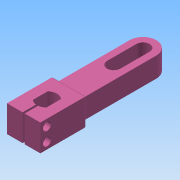
# Autodesk Inventor part: 刀轴拨叉
Saved by Autodesk Inventor 2015 (Build 190159000, 159)
## iProperties
Created: 2017-05-26
Part Number: 刀轴拨叉
Material: 常规
Document SubType Name: Modeling
Designer: Administrator
Density: 1 g/cm^3
Appearance: 粉红色
Author: Administrator
Autodesk Inventor part; units mm, degrees
ref_plane "YZ Plane" through (0, 0, 0) normal (1, 0, 0) x (0, 1, 0)
ref_plane "XZ Plane" through (0, 0, 0) normal (0, 1, 0) x (-1, 0, 0)
ref_plane "XY Plane" through (0, 0, 0) normal (0, 0, 1) x (1, 0, 0)
sketch "草图1" plane through (0, 0, 0) normal (0, 0, 1) x (1, 0, 0)
  line L0 (-12.5, 17.5) -> (12.5, 17.5)
  line L1 (12.5, 17.5) -> (12.5, -17.5)
  line L2 (12.5, -17.5) -> (-12.5, -17.5)
  line L3 (-12.5, -17.5) -> (-12.5, 17.5)
  line L4 (0, 0) -> (12.5, 0)
  line L5 (0, 0) -> (0, 17.5)
  circle A0 centre (0, 0) radius 7.5
  line L6 (10, 17.5) -> (-10, 17.5)
  line L7 (-10, 17.5) -> (-10, 82)
  line L8 (-10, 82) -> (10, 82)
  line L9 (10, 82) -> (10, 17.5)
  point P0 (0, 82)
  dimension "d0" = 25
  dimension "d1" = 35
  dimension "d2" = 15
  dimension "d3" = 20
  dimension "d13" = 82
  constraints: 20 end point, 5 parallel, 3 horizontal, 3 midpoint, 2 perpendicular, 2 point on line, 1 centre point, 1 coincident
  measures "d0" distance of L1.end L2.end
  measures "d1" distance of L0.end L1.end
  measures "d2" diameter of A0
  measures "d3" distance of L7.end L8.end
  measures "d13" distance from line of L4.start L8
extrude "拉伸1" add sketch "草图1" along normal blind 20
sketch "草图2" plane through (0, 0, 20) normal (0, 0, 1) x (1, 0, 0)
  circle A0 centre (0, 0) radius 7.5
  line L0 (-12.5, -17.5) -> (12.5, -17.5) projected
  line L1 (-0.75, -7.4624) -> (0.75, -7.4624)
  line L2 (0.75, -7.4624) -> (0.75, -17.5)
  line L3 (0.75, -17.5) -> (-0.75, -17.5)
  line L4 (-0.75, -17.5) -> (-0.75, -7.4624)
  circle A1 centre (0, 72) radius 5
  circle A2 centre (0, 50) radius 5
  line L5 (10, 82) -> (-10, 82) projected
  line L6 (-5, 72) -> (-5, 50)
  line L7 (5, 72) -> (5, 50)
  line L8 (10, 17.5) -> (10, 82) projected
  dimension "d7" = 15
  dimension "d8" = 1.5
  dimension "d9" = 10
  dimension "d10" = 10
  dimension "d11" = 10
  dimension "d12" = 50
  dimension "d14" = 10
  constraints: 12 end point, 6 point on circle, 4 tangent, 3 centre point, 2 parallel, 1 coincident, 1 horizontal, 1 perpendicular, 1 point on line, 1 vertical
  measures "d7" diameter of A0
  measures "d8" distance between parallel lines of L2 L4
  measures "d9" diameter of A1
  measures "d10" diameter of A2
  measures "d11" distance from line of L5 A1.centre
  measures "d12" distance of point (0, 0) A2.centre
  measures "d14" distance from line of L8 A1.centre
extrude "拉伸2" cut sketch "草图2" against normal through all
sketch "草图3" plane through (10, 17.5, 0) normal (1, 0, 0) x (0, 0, -1)
  line L0 (0, 0) -> (-20, 0) projected
  line L1 (-20, 64.5) -> (-17.5, 64.5)
  line L2 (-17.5, 64.5) -> (-17.5, 0)
  line L3 (-17.5, 0) -> (-20, 0)
  line L4 (-20, 0) -> (-20, 64.5)
  line L5 (0, 64.5) -> (-2.5, 64.5)
  line L6 (-2.5, 64.5) -> (-2.5, 0)
  line L7 (-2.5, 0) -> (0, 0)
  line L8 (0, 0) -> (0, 64.5)
  point P0 (0, -17.5)
  dimension "d17" = 15
  dimension "d18" = 2.5
  constraints: 16 end point, 4 parallel, 2 horizontal, 2 perpendicular, 2 point on line
  measures "d17" distance between parallel lines of L6 L2
  measures "d18" distance between parallel lines of L4 L2
extrude "拉伸3" cut sketch "草图3" against normal through all
sketch "草图4" plane through (-12.5, -17.5, 0) normal (-1, 0, 0) x (0, 0, 1)
  circle A0 centre (5, 5) radius 1.5
  circle A1 centre (15, 5) radius 1.5
  line L0 (0, 0) -> (20, 0) projected
  line L1 (20, 35) -> (20, 0) projected
  line L2 (0, 35) -> (0, 0) projected
  point P0 (0, 17.5)
  dimension "d21" = 3
  dimension "d22" = 3
  dimension "d23" = 5
  dimension "d24" = 5
  dimension "d25" = 5
  dimension "d26" = 5
  constraints: 2 centre point
  measures "d21" diameter of A0
  measures "d22" diameter of A1
  measures "d23" distance from line of L0 A1.centre
  measures "d24" distance from line of L0 A0.centre
  measures "d25" distance from line of L1 A1.centre
  measures "d26" distance from line of L2 A0.centre
extrude "拉伸4" cut sketch "草图4" against normal through all
sketch "草图5" plane through (12.5, -17.5, 0) normal (1, 0, 0) x (0, 0, -1)
  circle A0 centre (-5, 5) radius 3
  circle A1 centre (-15, 5) radius 3
  circle A2 centre (-5, 5) radius 1.5 projected
  circle A3 centre (-15, 5) radius 1.5 projected
  point P0 (0, 17.5)
  dimension "d29" = 6
  dimension "d30" = 6
  constraints: 2 centre point, 2 concentric
  measures "d29" diameter of A0
  measures "d30" diameter of A1
extrude "拉伸5" cut sketch "草图5" against normal blind 4
thread "螺纹1" size "M3x0.5" class "6H" standard "ANSI Metric M Profile" full length
thread "螺纹2" size "M3x0.5" class "6H" standard "ANSI Metric M Profile" full length
sketch "草图6" plane through (0, 0, 0) normal (0, 0, -1) x (-1, 0, 0)
  line L0 (5, 5.5902) -> (5, -5.5902)
  line L1 (5, -5.5902) -> (-5, -5.5902)
  line L2 (-5, -5.5902) -> (-5, 5.5902)
  arc A0 (0.75, -7.4624) -> (-0.75, -7.4624) centre (0, 0) ccw projected
  arc A1 (-5, 5.5902) -> (-5, -5.5902) centre (0, 0) ccw
  arc A2 (5, -5.5902) -> (5, 5.5902) centre (0, 0) ccw
  dimension "d37" = 10
  dimension "d38" = 5.5902
  constraints: 7 point on circle, 6 end point, 3 concentric, 2 centre point, 2 parallel
  measures "d37" distance of L0.end L1.end
  measures "d38" vertical distance of L0.start point (0, 0)
extrude "拉伸6" add sketch "草图6" against normal blind 20 contours A0 L0 | L2 A0
fillet "圆角1" radius 10 2 edges at (10, 82, 10) (-10, 82, 10)
fillet "圆角2" radius 2 5 edges at (12.5, 17.5, 10) (10, 17.5, 10) (0, 17.5, 0) (-12.5, 17.5, 10) (0, 17.5, 20)
